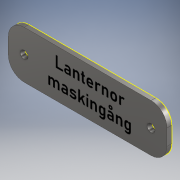
# Autodesk Inventor part: label
Saved by Autodesk Inventor 2019.2 (Build 232265000, 265)
## iProperties
Created: 2020-05-18
Part Number: label
Material: Stainless Steel
Document SubType Name: Modeling
Designer: Johansson
Density: 8 g/cm^3
Appearance: Semi-Polished
Author: Johansson
Autodesk Inventor part; units mm, degrees
ref_plane "YZ Plane" through (0, 0, 0) normal (1, 0, 0) x (0, 1, 0)
ref_plane "XZ Plane" through (0, 0, 0) normal (0, 1, 0) x (-1, 0, 0)
ref_plane "XY Plane" through (0, 0, 0) normal (0, 0, 1) x (1, 0, 0)
sketch "Sketch1" plane through (0, 0, 0) normal (0, 0, 1) x (1, 0, 0)
  line L0 (-25, -7.5) -> (25, -7.5)
  line L1 (25, -7.5) -> (25, 7.5)
  line L2 (25, 7.5) -> (-25, 7.5)
  line L3 (-25, 7.5) -> (-25, -7.5)
  line L4 (-25, -7.5) -> (25, 7.5) construction
  line L5 (25, -7.5) -> (-25, 7.5) construction
  point P0 (0, 0)
  dimension "d0" = 50
  dimension "d1" = 15
  constraints: 12 end point, 2 midpoint, 2 parallel, 1 horizontal, 1 perpendicular
  measures "d0" distance of L1.end L2.end
  measures "d1" distance of L2.end L0.start
extrude "Extrusion1" add sketch "Sketch1" along normal blind 1.5
sketch "Sketch2" plane through (0, 0, 1.5) normal (0, 0, 1) x (1, 0, 0)
  circle A0 centre (-20, 0) radius 1.25
  line L0 (0, -11.9497) -> (0, 11.9497) projected
  circle A1 centre (20, 0) radius 1.25
  line L1 (-25, 7.5) -> (-25, -7.5) projected
  point P0 (0, 0)
  dimension "d4" = 2.5
  dimension "d5" = 5
  constraints: 2 centre point, 1 symmetric about line, 1 other
  measures "d4" diameter of A0
  measures "d5" distance from line of L1 A0.centre
extrude "Extrusion2" cut sketch "Sketch2" against normal up to next
fillet "Fillet1" radius 5 4 edges at (25, 7.5, 0.75) (25, -7.5, 0.75) (-25, -7.5, 0.75) (-25, 7.5, 0.75)
sketch "Sketch3" plane through (0, 0, 1.5) normal (0, 0, 1) x (1, 0, 0)
  line L0 (-10.4543, 4.2971) -> (11.6893, 4.2971) construction
  line L1 (11.6893, 4.2971) -> (11.6893, -4.6339) construction
  line L2 (11.6893, -4.6339) -> (-10.4543, -4.6339) construction
  line L3 (-10.4543, -4.6339) -> (-10.4543, 4.2971) construction
  constraints: 2 other
sketch "Sketch4" plane through (0, 0, 0) normal (0, 0, -1) x (-1, 0, 0)
  line L0 (-10.4543, 4.2971) -> (11.6893, 4.2971) construction
  line L1 (11.6893, 4.2971) -> (11.6893, -4.6339) construction
  line L2 (11.6893, -4.6339) -> (-10.4543, -4.6339) construction
  line L3 (-10.4543, -4.6339) -> (-10.4543, 4.2971) construction
  constraints: 2 other
sketch "Sketch5" plane through (0, 0, 0) normal (0, 0, -1) x (-1, 0, 0)
  circle A0 centre (20, 0) radius 1.25 projected
  circle A1 centre (-20, 0) radius 1.25 projected
  arc A2 (25, 2.5) -> (20, 7.5) centre (20, 2.5) ccw projected
  line L0 (-20, 7.5) -> (20, 7.5) projected
  arc A3 (-20, 7.5) -> (-25, 2.5) centre (-20, 2.5) ccw projected
  line L1 (-25, -2.5) -> (-25, 2.5) projected
  arc A4 (-25, -2.5) -> (-20, -7.5) centre (-20, -2.5) ccw projected
  line L2 (20, -7.5) -> (-20, -7.5) projected
  arc A5 (20, -7.5) -> (25, -2.5) centre (20, -2.5) ccw projected
  line L3 (25, 2.5) -> (25, -2.5) projected
  point P0 (0, 0)
equation "\"d0\" = l_label"
equation "\"d1\" = w_label"
equation "\"d4\" = r_labelscrew"
equation "\"d5\" = ro_labelscrew"
equation "\"d8\" = ro_labelscrew"
equation "\"wl_panel\" = 265"
equation "\"t_panel\" = 8"
equation "\"r_button\" = 8"
equation "\"l_stereo\" = 178"
equation "\"d_stereo\" = 177"
equation "\"w_label\" = 15"
equation "\"l_label\" = 50"
equation "\"r_labelscrew\" = 2.5"
equation "\"ro_labelscrew\" = 5"
equation "\"l_buttontobutton\" = 25"
equation "\"r_usboutlet\" = 29"
equation "\"l_fastener_button\" = 19"
body "Solid1"
